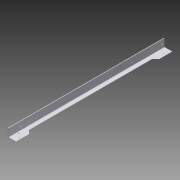
# Autodesk Inventor part: rail support 2x2 angle
Saved by Autodesk Inventor 2015 (Build 190159000, 159)
## iProperties
Created: 2015-01-26
Part Number: rail support 2x2 angle
Material: Aluminum 6061
Document SubType Name: Modeling
Designer: Admin
Density: 2.7 g/cm^3
Appearance: Aluminum - Flat
Author: Admin
Autodesk Inventor part; units mm, degrees
ref_plane "YZ Plane" through (0, 0, 0) normal (1, 0, 0) x (0, 1, 0)
ref_plane "XZ Plane" through (0, 0, 0) normal (0, 1, 0) x (-1, 0, 0)
ref_plane "XY Plane" through (0, 0, 0) normal (0, 0, 1) x (1, 0, 0)
sketch "Sketch1" plane through (0, 0, 0) normal (0, 0, 1) x (1, 0, 0)
  line L0 (0, 0) -> (3.175, 0)
  line L1 (3.175, 0) -> (3.175, 50.8)
  line L2 (3.175, 50.8) -> (0, 50.8)
  line L3 (0, 50.8) -> (0, 0)
  line L4 (0, 0) -> (50.8, 0)
  line L5 (50.8, 0) -> (50.8, 3.175)
  line L6 (50.8, 3.175) -> (0, 3.175)
  line L7 (0, 3.175) -> (0, 0)
  dimension "d0" = 3.175
  dimension "d1" = 50.8
  dimension "d2" = 50.8
  dimension "d3" = 3.175
  constraints: 16 end point, 4 parallel, 2 horizontal, 2 perpendicular
  measures "d0" distance of L2.end L1.end
  measures "d1" distance of L1.end L0.end
  measures "d2" distance of L6.end L5.end
  measures "d3" distance of L5.end L4.end
extrude "Extrusion1" add sketch "Sketch1" along normal blind 965.2
sketch "Sketch2" plane through (0, 0, 0) normal (-1, 0, 0) x (0, 0, 1)
  line L0 (0, 50.8) -> (0, 0) projected
  line L1 (0, 0) -> (965.2, 0) projected
  point P0 (12.7, 23.8125)
  point P1 (203.2, 23.8125)
  dimension "d6" = 23.8125
  dimension "d7" = 23.8125
  dimension "d8" = 12.7
  dimension "d9" = 203.2
  measures "d6" distance from line of L1 point (12.7, 23.812)
  measures "d7" distance from line of L1 point (203.2, 23.812)
  measures "d8" distance from line of L0 point (12.7, 23.812)
  measures "d9" distance from line of L0 point (203.2, 23.812)
hole "Hole1" at (0, 23.8125, 12.7) at (0, 23.8125, 203.2) direction (1, 0, 0) diameter 6.35 end through all
sketch "Sketch3" plane through (0, 0, 0) normal (-1, 0, 0) x (0, 0, 1)
  line L0 (0, 0) -> (965.2, 0) projected
  line L1 (0, 50.8) -> (0, 0) projected
  point P0 (889, 23.8125)
  dimension "d17" = 23.8125
  dimension "d26" = 889
  measures "d17" distance from line of L0 point (889, 23.812)
  measures "d26" distance from line of L1 point (889, 23.812)
hole "Hole2" at (0, 23.8125, 889) direction (1, 0, 0) diameter 9.525 end through all
sketch "Sketch4" plane through (0, 0, 0) normal (0, -1, 0) x (1, 0, 0)
  line L0 (0, 965.2) -> (50.8, 965.2) projected
  line L1 (0, 0) -> (0, 965.2) projected
  point P0 (17.4625, 914.4)
  dimension "d27" = 17.4625
  dimension "d28" = 50.8
  measures "d27" distance from line of L1 point (17.463, 914.4)
  measures "d28" distance from line of L0 point (17.463, 914.4)
hole "Hole3" at (17.4625, 0, 914.4) direction (0, 1, 0) diameter 6.35 end through all
fillet "Fillet1" radius 3.175 1 edges at (3.175, 3.175, 482.6)
sketch "Sketch6" plane through (0, 0, 0) normal (0, -1, 0) x (1, 0, 0)
  line L0 (0, 0) -> (50.8, 0) projected
  line L1 (50.8, 0) -> (50.8, 965.2) projected
  line L2 (0, 965.2) -> (50.8, 965.2) projected
  point P0 (38.1, 933.45)
  point P1 (38.1, 38.1)
  dimension "d49" = 38.1
  dimension "d50" = 12.7
  dimension "d51" = 31.75
  dimension "d52" = 12.7
  measures "d49" distance from line of L0 point (38.1, 38.1)
  measures "d50" distance from line of L1 point (38.1, 38.1)
  measures "d51" distance from line of point (38.1, 933.45) L2
  measures "d52" distance from line of L1 point (38.1, 933.45)
hole "Hole5" at (38.1, 0, 933.45) at (38.1, 0, 38.1) direction (0, 1, 0) diameter 4.7625 end through all
sketch "Sketch8" plane through (0, 0, 0) normal (0, -1, 0) x (1, 0, 0)
  circle A0 centre (38.1, 933.45) radius 2.3813 projected
  circle A1 centre (38.1, 38.1) radius 2.3813 projected
  circle A2 centre (17.4625, 914.4) radius 3.175 projected
  line L0 (0, 0) -> (50.8, 0) projected
  line L1 (50.8, 0) -> (50.8, 965.2) projected
  line L2 (0, 965.2) -> (50.8, 965.2) projected
  line L3 (0, 0) -> (0, 965.2) projected
  line L4 (50.8, 863.6) -> (28.575, 863.6)
  line L5 (28.575, 863.6) -> (28.575, 101.6)
  line L6 (28.575, 101.6) -> (50.8, 101.6)
  line L7 (50.8, 101.6) -> (50.8, 863.6)
  line L8 (28.575, 863.6) -> (50.8, 885.825)
  line L9 (50.8, 0) -> (50.8, 965.2) projected
  line L10 (28.575, 863.6) -> (60.0059, 863.6) construction
  line L11 (50.8, 885.825) -> (50.8, 863.6)
  line L12 (28.575, 101.6) -> (50.8, 79.375)
  line L13 (28.575, 101.6) -> (60.0059, 101.6) construction
  line L14 (50.8, 79.375) -> (50.8, 101.6)
  dimension "d60" = 22.225
  dimension "d61" = 101.6
  dimension "d62" = 101.6
  dimension "d63" = 45
  dimension "d64" = 45
  constraints: 20 end point, 3 horizontal, 3 point on line, 2 collinear, 2 equal length, 2 parallel, 1 perpendicular
  measures "d60" distance of L6.end L5.end
  measures "d61" distance between parallel lines of L0 L6
  measures "d62" distance between parallel lines of L2 L4
  measures "d63" angle of L10 L8
  measures "d64" angle of L12 L13
extrude "Extrusion2" cut sketch "Sketch8" against normal blind 25.4 contours L12 L6 L1 | L6 L5 L4 L1 | L1 L4 L8
sketch "Sketch9" plane through (0, 0, 0) normal (-1, 0, 0) x (0, 0, 1)
  circle A0 centre (889, 23.8125) radius 4.7625 projected
  circle A1 centre (12.7, 23.8125) radius 3.175 projected
  circle A2 centre (203.2, 23.8125) radius 3.175 projected
  line L0 (0, 50.8) -> (0, 0) projected
  line L1 (0, 0) -> (965.2, 0) projected
  line L2 (965.2, 50.8) -> (965.2, 0) projected
  line L3 (0, 50.8) -> (965.2, 50.8) projected
  point P0 (838.2, 23.8125)
  dimension "d67" = 23.8125
  dimension "d68" = 127
  measures "d67" distance from line of L1 point (838.2, 23.812)
  measures "d68" distance from line of L2 point (838.2, 23.812)
hole "Hole6" at (0, 23.8125, 838.2) direction (1, 0, 0) diameter 6.35 end through all
body "Solid1"
